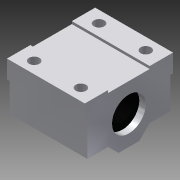
# Autodesk Inventor part: Linear Bearing Platform Small
Saved by Autodesk Inventor 2015 SP1 (Build 190203100, 203)
## iProperties
Created: 2015-02-23
Part Number: Linear Bearing Platform Small
Material: Aluminum 6061
Document SubType Name: Modeling
Designer: Andrew
Density: 2.7 g/cm^3
Appearance: Aluminum - Flat
Author: Andrew
Autodesk Inventor part; units mm, degrees
ref_plane "YZ Plane" through (0, 0, 0) normal (1, 0, 0) x (0, 1, 0)
ref_plane "XZ Plane" through (0, 0, 0) normal (0, 1, 0) x (-1, 0, 0)
ref_plane "XY Plane" through (0, 0, 0) normal (0, 0, 1) x (1, 0, 0)
sketch "Sketch1" plane through (0, 0, 0) normal (1, 0, 0) x (0, 1, 0)
  circle A0 centre (0, 0) radius 4
  line L0 (0, 23.8) -> (0, -23.8) projected
  line L1 (-15.6, 0) -> (16.6, 0) projected
  line L2 (11, 17) -> (11, -17)
  line L3 (11, -17) -> (5, -17)
  line L4 (5, -17) -> (5, -16)
  line L5 (5, -16) -> (-7, -16)
  line L6 (-7, -16) -> (-7, -8)
  line L7 (-7, -8) -> (-11, -4)
  line L8 (-11, -4) -> (-11, 4)
  line L9 (-11, 4) -> (-7, 8)
  line L10 (-7, 8) -> (-7, 16)
  line L11 (-7, 16) -> (5, 16)
  line L12 (5, 16) -> (5, 17)
  line L13 (5, 17) -> (11, 17)
  circle A1 centre (0, 0) radius 6.5
  line L14 (11, -12) -> (-7, -12) construction
  line L15 (-7, -14) -> (11, -14) construction
  line L16 (11, -10) -> (-7, -10) construction
  line L17 (11, -17) -> (12, -17)
  line L18 (12, -17) -> (12, -8)
  line L19 (12, -8) -> (11, -8)
  line L20 (11, 17) -> (12, 17)
  line L21 (12, 17) -> (12, 8)
  line L22 (12, 8) -> (11, 8)
  dimension "d0" = 34
  dimension "d1" = 22
  dimension "d2" = 11
  dimension "d3" = 6
  dimension "d4" = 18
  dimension "d5" = 1
  dimension "d6" = 8
  dimension "d7" = 13
  dimension "d9" = 5
  dimension "d10" = 4
  dimension "d11" = 4
  dimension "d12" = 8
  dimension "d17" = 1
  constraints: 42 end point, 12 perpendicular, 12 point on line, 2 centre point, 2 coincident, 2 horizontal, 2 parallel, 1 midpoint, 1 vertical, 8 other
  measures "d0" distance between parallel lines of L3 L13
  measures "d1" distance between parallel lines of L8 L2
  measures "d2" distance from line of L2 point (0, 0)
  measures "d3" distance between parallel lines of L2 L4
  measures "d4" distance between parallel lines of L10 L2
  measures "d5" distance between parallel lines of L3 L5
  measures "d6" diameter of A0
  measures "d7" diameter of A1
  measures "d9" distance between parallel lines of L3 L14
  measures "d10" distance of L6.end L14.end
  measures "d11" distance between parallel lines of L15 L16
  measures "d12" distance of L7.end L8.end
  measures "d17" distance between parallel lines of L2 L18
extrude "Extrusion1" add sketch "Sketch1" along normal mid plane 30 contours A1 L0 L11 L12 L13 L2 L1 | L1 L2 L3 L4 L5 L0 A1 | A1 L1 L8 L9 L10 L11 L0 | L0 L5 L6 L7 L8 L1 A1 | L2 L20 L21 L22 | L19 L18 L17 L2
extrude "Extrusion2" add sketch "Sketch1" along normal mid plane 25 contours L1 A1 L0 A0 | A0 L0 A1 L1 | A0 L1 A1 L0 | L0 A1 L1 A0
sketch "Sketch2" plane through (-15, 12, 17) normal (0, 1, 0) x (1, 0, 0)
  line L0 (30, 0) -> (0, 0) projected
  line L1 (30, 9) -> (30, 0) projected
  line L2 (0, 9) -> (30, 9) projected
  line L3 (0, 0) -> (0, 9) projected
  line L4 (0, 25) -> (30, 25) projected
  line L5 (30, 34) -> (30, 25) projected
  line L6 (0, 34) -> (30, 34) projected
  line L7 (0, 25) -> (0, 34) projected
  line L8 (36, 17) -> (-6, 17) projected
  line L9 (15, 40.8) -> (15, -6.8) projected
  circle A0 centre (6, 4.5) radius 2
  circle A1 centre (24, 4.5) radius 2
  circle A2 centre (6, 29.5) radius 2
  circle A3 centre (24, 29.5) radius 2
  point P0 (15, 17)
  dimension "d18" = 4.5
  dimension "d19" = 18
  dimension "d20" = 4
  constraints: 4 centre point, 4 other
  measures "d18" distance from line of A0.centre L0
  measures "d19" distance of A1.centre A0.centre
  measures "d20" diameter of A0
extrude "Extrusion3" cut sketch "Sketch2" against normal up to next contours A0 | A1 | A2 | A3
body "Solid1"
